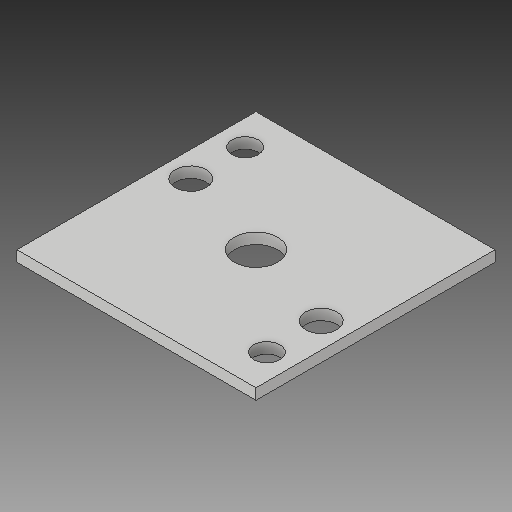
# Autodesk Inventor part: Luxcan P1
Saved by Autodesk Inventor 2018 (Build 220112000, 112)
## iProperties
Created: 2018-07-26
Part Number: Luxcan P1
Material: Generic
Document SubType Name: Sheet Metal
Designer: jocdurso
Density: 1 g/cm^3
Sheet Metal Rule: Default
Appearance: Default
Author: jocdurso
Autodesk Inventor part; units mm, degrees
ref_plane "YZ Plane" through (0, 0, 0) normal (1, 0, 0) x (0, 1, 0)
ref_plane "XZ Plane" through (0, 0, 0) normal (0, 1, 0) x (-1, 0, 0)
ref_plane "XY Plane" through (0, 0, 0) normal (0, 0, 1) x (1, 0, 0)
sketch "Sketch1" plane through (0, 0, 0) normal (0, 1, 0) x (-1, 0, 0)
  line L0 (16.5, -16.5) -> (-16.5, -16.5)
  line L1 (-16.5, -16.5) -> (-16.5, 16.5)
  line L2 (-16.5, 16.5) -> (16.5, 16.5)
  line L3 (16.5, 16.5) -> (16.5, -16.5)
  point P0 (0, 0)
  point P1 (16.5, 0)
  point P2 (0, -16.5)
  dimension "d0" = 33
  dimension "d1" = 33
  measures "d0" distance of L0.start L0.end
  measures "d1" distance of L2.end L0.start
extrude "Plate1" add sketch "Sketch1" along normal blind 1.5
sketch "Sketch2" plane through (0, 0, 0) normal (0, 1, 0) x (-1, 0, 0)
  point P0 (0, 0)
  point P1 (0, 0)
  constraints: 1 coincident
hole "Hole1" at (0, 0, 0) direction (0, 1, 0) diameter 6 end through all
sketch "Sketch3" plane through (0, 0, 0) normal (0, 1, 0) x (-1, 0, 0)
  line L0 (0, 0) -> (0, -16.3603)
  point P0 (13, -4)
  point P1 (-13, 4)
  dimension "d10" = 4
  dimension "d11" = 13
  dimension "d12" = 4
  dimension "d13" = 13
  constraints: 2 end point, 1 vertical
  measures "d10" vertical distance of point (13, -4) L0.start
  measures "d11" horizontal distance of L0.start point (13, -4)
  measures "d12" vertical distance of L0.start point (-13, 4)
  measures "d13" horizontal distance of L0.start point (-13, 4)
hole "Hole2" at (-13, 0, -4) at (13, 0, 4) direction (0, 1, 0) diameter 4.3 end through all
sketch "Sketch4" plane through (0, 0, 0) normal (0, 1, 0) x (-1, 0, 0)
  point P0 (0, 0)
  point P1 (13, -11.5)
  point P2 (-13, 11.5)
  dimension "d21" = 13
  dimension "d22" = 11.5
  dimension "d23" = 11.5
  dimension "d24" = 13
  measures "d21" horizontal distance of point (0, 0) point (13, -11.5)
  measures "d22" vertical distance of point (0, 0) point (13, -11.5)
  measures "d23" vertical distance of point (-13, 11.5) point (0, 0)
  measures "d24" horizontal distance of point (0, 0) point (-13, 11.5)
hole "Hole3" at (-13, 0, -11.5) at (13, 0, 11.5) direction (0, 1, 0) diameter 3.6 end through all
equation "\"d8\" = Thickness"
equation "\"d19\" = Thickness"
equation "\"d30\" = Thickness"
equation "\"d32\" = Thickness"
equation "\"BendRadius\" = Thickness"
equation "\"BendReliefWidth\" = Thickness"
equation "\"BendReliefDepth\" = 0.5 * Thickness"
equation "\"CornerReliefSize\" = 4 * Thickness"
equation "\"MinimumRemnant\" = 2 * Thickness"
equation "\"TransitionRadius\" = BendRadius"
equation "\"JacobiRadiusSize\" = BendRadius"
equation "\"GapSize\" = Thickness"
equation "\"d2\" = BendRadius"
equation "\"Thickness\" = 1.5"
body "Solid1"
